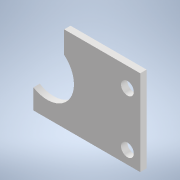
# Autodesk Inventor part: domePlaceSingle
Saved by Autodesk Inventor 2022 (Build 260153000, 153)
## iProperties
Created: 2021-07-01
Part Number: domePlaceSingle
Material: Generic
Document SubType Name: Modeling
Designer: dsdan
Density: 1 g/cm^3
Appearance: Default
Author: dsdan
Autodesk Inventor part; units mm, degrees
ref_plane "YZ Plane" through (0, 0, 0) normal (1, 0, 0) x (0, 1, 0)
ref_plane "XZ Plane" through (0, 0, 0) normal (0, 1, 0) x (-1, 0, 0)
ref_plane "XY Plane" through (0, 0, 0) normal (0, 0, 1) x (1, 0, 0)
sketch "Sketch1" plane through (0, 0, 0) normal (0, 0, 1) x (1, 0, 0)
  circle A0 centre (0, 0) radius 12.5
  line L0 (-43.5003, 20.018) -> (43.5003, 20.018)
  line L1 (43.5003, 20.018) -> (43.5003, -20.018)
  line L2 (43.5003, -20.018) -> (-43.5003, -20.018)
  line L3 (-43.5003, -20.018) -> (-43.5003, 20.018) construction
  line L4 (-43.5003, 20.018) -> (43.5003, -20.018) construction
  line L5 (43.5003, 20.018) -> (-43.5003, -20.018) construction
  line L6 (7.8932, 9.6927) -> (7.8932, 20.018)
  line L7 (-6.4997, -10.6772) -> (-6.4997, -20.018)
  circle A1 centre (37.5003, 10.982) radius 3.5 construction
  circle A2 centre (37.5003, -14.018) radius 3.5 construction
  circle A3 centre (37.5003, 10.982) radius 3
  circle A4 centre (37.5003, -14.018) radius 3
  dimension "d0" = 25
  dimension "d6" = 50
  dimension "d7" = 6
  dimension "d8" = 6
  dimension "d9" = 6
  dimension "d10" = 6
  constraints: 16 end point, 3 centre point, 3 coincident, 3 perpendicular, 2 midpoint, 2 parallel, 2 point on circle, 2 point on line, 1 horizontal
  measures "d0" diameter of A0
  measures "d6" distance between parallel lines of L1 L7
  measures "d7" diameter of A3
  measures "d8" diameter of A4
  measures "d9" distance from line of A3.centre L1
  measures "d10" distance from line of A4.centre L2
extrude "Extrusion1" add sketch "Sketch1" along normal blind 3 contours A0 L6 L0 L1 L2 L7
body "Solid1"
